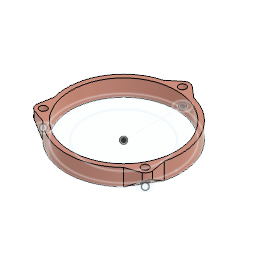
RingTop (Autodesk Fusion 360 design; units mm, degrees)
Autodesk Fusion 360 part; units mm, degrees
sketch "Sketch2" plane through (0, 0, 0) normal (0, 0, 1) x (1, 0, 0)
  circle A0 centre (0, 0) radius 34
  circle A1 centre (0, 0) radius 22.5
  circle A2 centre (0, 0) radius 31.25
  line L0 (0, 0) -> (0, 35) construction
  circle A3 centre (0, 35) radius 2.15
  circle A4 centre (0, 35) radius 4.15
  circle A5 centre (-30.3109, -17.5) radius 4.15
  circle A6 centre (-30.3109, -17.5) radius 2.15
  circle A7 centre (30.3109, -17.5) radius 4.15
  circle A8 centre (30.3109, -17.5) radius 2.15
  dimension "d19" = 68
  dimension "d21" = 45
  dimension "d29" = 62.5
  dimension "d75" = 35
  dimension "d76" = 4.3
  dimension "d78" = 2
  dimension "d80" = 360
  constraint coincident A0.centre A1.centre
  constraint concentric A0 A1
  constraint concentric A0 A2
  constraint vertical L0
  constraint coincident L0.end A3.centre
  measures "d19" diameter of A0
  measures "d21" diameter of A1
  measures "d29" diameter of A2
  measures "d75" distance of A0.centre L0.end
  measures "d76" diameter of A3
extrude "main" add sketch "Sketch2" along normal blind 10 contours A0 A2 A4 A7 | A0 A2 A3 A4 | A0 A3 A4 | A0 A7 A8 | A0 A2 A7 A8 | A0 A2 A4 A5 | A0 A2 A5 A7 | A0 A2 A5 A6 | A0 A5 A6
chamfer "Chamfer4" distance 5 angle 45 6 edges at (31.2257, -13.4521, 5) (3.963, 33.7683, 5) (-3.963, 33.7683, 5) (-31.2257, -13.4521, 5) (-27.2627, -20.3162, 5) (27.2627, -20.3162, 5)
sketch "Sketch4" plane through (0, 0, 0) normal (1, 0, 0) x (0, 1, 0)
  line L0 (0, 0) -> (33, 0) construction
  line L1 (33, 0) -> (49.4315, 16.4315)
  line L2 (33, 0) -> (56.2377, 0)
  line L3 (49.4315, 16.4315) -> (49.4315, 0)
  dimension "d69" = 33
  dimension "d70" = 45
  constraint horizontal L0
  constraint coincident L0.start origin
  constraint horizontal L2
  constraint coincident L2 L3.end
  constraint perpendicular L2 L3
  measures "d69" distance of L0.start L0.end
  measures "d70" angle of L1 L2
extrude "Extrude8" cut sketch "Sketch4" along normal mid plane 20
pattern_circular "C-Pattern3" count 3 over 360 about axis through (0, 0, 1.75) along (0, 0, 1) of "Extrude8"
equation "gear_ratio = 6"
equation "gear_Ns = if(is_Nema_17 == 1; 12; 15)"
equation "gear_Nr = ( gear_ratio - 1 ) * gear_Ns"
equation "gear_OD = ( gear_Nr * diameter_scale * module ) + 8 mm"
equation "ring_width = 52 mm"
equation "m3_hole_thickness = 2 mm"
equation "m3_inserts = 4.3 mm"
equation "d19 = gear_OD"
equation "output_bearing_od = 47 mm"
equation "d21 = output_bearing_od - 2 mm"
equation "d29 = gear_OD - wall_thickness + 1.5 mm"
equation "wall_thickness = 7 mm"
equation "d33 = height"
equation "height = 10 mm"
equation "module = 1"
equation "helix_angle = 0 deg"
equation "diameter_scale = ( 1 / cos(helix_angle) ) * 1 mm"
equation "d69 = ( gear_OD / 2 ) - 1 mm"
equation "d75 = ( gear_OD / 2 ) + 1 mm"
equation "d76 = m3_inserts"
equation "d78 = m3_hole_thickness"
equation "is_Nema_17 = 1"
